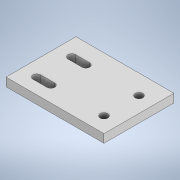
# Autodesk Inventor part: Y_Carriage_Plate
Saved by Autodesk Inventor 2021 (Build 250183000, 183)
## iProperties
Created: 2021-06-15
Part Number: Y_Carriage_Plate
Material: Generic
Document SubType Name: Modeling
Designer: Jorian Brusind
Density: 1 g/cm^3
Appearance: Default
Author: Jorian Brusind
Autodesk Inventor part; units mm, degrees
ref_plane "YZ Plane" through (0, 0, 0) normal (1, 0, 0) x (0, 1, 0)
ref_plane "XZ Plane" through (0, 0, 0) normal (0, 1, 0) x (-1, 0, 0)
ref_plane "XY Plane" through (0, 0, 0) normal (0, 0, 1) x (1, 0, 0)
sketch "Sketch1" plane through (0, 0, 0) normal (0, 1, 0) x (-1, 0, 0)
  line L0 (0, 0) -> (70, 0)
  line L1 (70, 0) -> (70, -50)
  line L2 (70, -50) -> (0, -50)
  line L3 (0, -50) -> (0, 0)
  dimension "d0" = 70
  dimension "d1" = 50
  constraints: 8 end point, 2 parallel, 1 horizontal, 1 perpendicular
  measures "d0" distance of L1.end L2.end
  measures "d1" distance of L0.end L1.end
extrude "Extrusion1" add sketch "Sketch1" along normal blind 6
sketch "Sketch2" plane through (0, 6, 0) normal (0, 1, 0) x (1, 0, 0)
  circle A0 centre (-11, 11) radius 2.75
  line L0 (0, 0) -> (0, 50) projected
  line L1 (-70, 0) -> (0, 0) projected
  dimension "d4" = 5.5
  dimension "d5" = 11
  dimension "d6" = 11
  constraints: 1 centre point
  measures "d4" diameter of A0
  measures "d5" distance from line of L0 A0.centre
  measures "d6" distance from line of L1 A0.centre
extrude "Extrusion2" cut sketch "Sketch2" against normal through all
pattern_linear "Rectangular Pattern1" count 2 spacing 38 along (-1, 0, 0) count 2 spacing 25 along (0, 0, -1) of "Extrusion2"
sketch "Sketch3" plane through (0, 6, 0) normal (0, 1, 0) x (1, 0, 0)
  circle A0 centre (-49, 11) radius 2.75 projected
  line L0 (-49, 11) -> (-59, 11) construction
  line L1 (-49, 13.75) -> (-59, 13.75)
  line L2 (-59, 8.25) -> (-49, 8.25)
  arc A1 (-49, 8.25) -> (-49, 13.75) centre (-49, 11) ccw
  arc A2 (-59, 13.75) -> (-59, 8.25) centre (-59, 11) ccw
  circle A3 centre (-49, 36) radius 2.75 projected
  line L3 (-49, 36) -> (-59, 36) construction
  line L4 (-49, 38.75) -> (-59, 38.75)
  line L5 (-59, 33.25) -> (-49, 33.25)
  arc A4 (-49, 33.25) -> (-49, 38.75) centre (-49, 36) ccw
  arc A5 (-59, 38.75) -> (-59, 33.25) centre (-59, 36) ccw
  point P0 (0, 0)
  point P1 (-54, 11)
  point P2 (-54, 36)
  dimension "d15" = 10
  dimension "d16" = 5.5
  dimension "d17" = 10
  dimension "d18" = 5.5
  constraints: 16 end point, 8 point on circle, 8 tangent, 4 centre point, 3 parallel, 2 midpoint, 1 horizontal
  measures "d15" distance of L0.start L0.end
  measures "d16" diameter of A2
  measures "d17" distance of L3.start L3.end
  measures "d18" diameter of A5
extrude "Extrusion3" cut sketch "Sketch3" against normal through all
body "Solid1"
